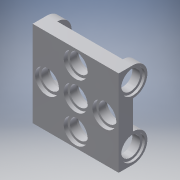
# Autodesk Inventor part: OlloHubToBase
Saved by Autodesk Inventor 2017 (Build 210142000, 142)
## iProperties
Created: 2016-06-20
Part Number: OlloHubToBase
Material: Generic
Document SubType Name: Modeling
Designer: Labtech
Density: 1 g/cm^3
Appearance: White
Author: Labtech
Autodesk Inventor part; units mm, degrees
note: some values were not read from the file. Chosen so that the rebuilt part matches the saved one: second side of "Extrusion7".
ref_plane "YZ Plane" through (0, 0, 0) normal (1, 0, 0) x (0, 1, 0)
sketch "Sketch1" plane through (0, 0, 0) normal (0, 1, 0) x (-1, 0, 0)
  line L0 (-9, 9) -> (9, 9)
  line L1 (9, 9) -> (9, -9)
  line L2 (9, -9) -> (-9, -9)
  line L3 (-9, -9) -> (-9, 9)
  line L4 (-9, 9) -> (9, -9) construction
  line L5 (9, 9) -> (-9, -9) construction
  circle A0 centre (0, 0) radius 2
  line L6 (0, 0) -> (0, -6) construction
  circle A1 centre (0, -6) radius 2
  circle A2 centre (6, 0) radius 2
  circle A3 centre (0, 6) radius 2
  circle A4 centre (-6, 0) radius 2
  dimension "d0" = 18
  dimension "d1" = 18
  dimension "d2" = 4
  dimension "d3" = 6
  dimension "d8" = 4
  dimension "d11" = 360
  constraints: 14 end point, 5 centre point, 2 coincident, 2 midpoint, 2 parallel, 1 horizontal, 1 perpendicular, 1 vertical, 9 other
  measures "d0" distance of L1.end L2.end
  measures "d1" distance of L0.end L1.end
  measures "d2" diameter of A0
  measures "d3" distance of L6.start L6.end
  measures "d8" diameter of A1
extrude "Extrusion1" add sketch "Sketch1" along normal blind 3
sketch "Sketch2" plane through (0, 3, 0) normal (0, 1, 0) x (1, 0, 0)
  circle A0 centre (0, 6) radius 2 projected
  circle A1 centre (0, 0) radius 2.5
  circle A2 centre (0, 6) radius 2.5
  circle A3 centre (-6, 0) radius 2.5
  circle A4 centre (0, -6) radius 2.5
  circle A5 centre (6, 0) radius 2.5
  dimension "d15" = 5
  dimension "d16" = 5
  dimension "d19" = 360
  constraints: 5 centre point, 2 coincident, 9 other
  measures "d15" diameter of A1
  measures "d16" diameter of A2
extrude "Extrusion2" cut sketch "Sketch2" against normal blind 0.8
sketch "Sketch3" plane through (0, 0, 0) normal (0, -1, 0) x (1, 0, 0)
  circle A0 centre (0, 0) radius 2.5
  circle A1 centre (0, -6) radius 2.5 projected
  circle A2 centre (0, -6) radius 2.5
  circle A3 centre (6, 0) radius 2.5
  circle A4 centre (0, 6) radius 2.5
  circle A5 centre (-6, 0) radius 2.5
  dimension "d25" = 360
  constraints: 5 centre point, 2 coincident, 1 concentric, 9 other
extrude "Extrusion3" cut sketch "Sketch3" against normal blind 0.8
sketch "Sketch4" plane through (9, 0, 9) normal (1, 0, 0) x (0, 0, -1)
  line L0 (0, 3) -> (3, 3) construction
  line L1 (0, 3) -> (18, 3) projected
  circle A0 centre (3, 3) radius 3
  point P0 (9, 0)
  dimension "d29" = 3
  constraints: 2 end point, 1 coincident, 1 horizontal alignment, 1 point on line, 2 other
  measures "d29" distance of L0.start L0.end
extrude "Extrusion4" add sketch "Sketch4" against normal blind 2.15
sketch "Sketch5" plane through (9, 0, 9) normal (1, 0, 0) x (0, 0, -1)
  line L0 (0, 3) -> (6, 3) projected
  arc A0 (6, 3) -> (0, 3) centre (3, 3) ccw projected
  circle A1 centre (3, 3) radius 2
  point P0 (9, 0)
  dimension "d32" = 4
  constraints: 1 centre point, 1 coincident
  measures "d32" diameter of A1
extrude "Extrusion5" cut sketch "Sketch5" against normal blind 3 contours A1 L0 | L0 A1
sketch "Sketch6" plane through (9, 0, 9) normal (1, 0, 0) x (0, 0, -1)
  circle A0 centre (3, 3) radius 2 projected
  circle A1 centre (3, 3) radius 2.5
  point P0 (9, 0)
  dimension "d35" = 5
  constraints: 1 centre point, 1 coincident
  measures "d35" diameter of A1
extrude "Extrusion6" cut sketch "Sketch6" against normal blind 0.5
sketch "Sketch7" plane through (6.85, 0, 9) normal (-1, 0, 0) x (0, 0, 1)
  arc A0 (-1, 3) -> (-5, 3) centre (-3, 3) ccw projected
  circle A1 centre (-3, 3) radius 2.5
  point P0 (-9, 0)
  dimension "d38" = 5
  constraints: 1 centre point, 1 coincident
  measures "d38" diameter of A1
extrude "Extrusion7" cut sketch "Sketch7" along normal blind 1
ref_plane "Work Plane1" through (-9, 0, 0) normal (0, 0, 1) x (1, 0, 0)
ref_plane "Work Plane2" through (0, 0, -9) normal (-1, 0, 0) x (0, 0, 1)
mirror "Mirror1" about plane through (-9, 0, 0) normal (0, 0, 1) of "Extrusion4", "Extrusion5", "Extrusion6", "Extrusion7"
mirror "Mirror2" about plane through (0, 0, -9) normal (-1, 0, 0) of "Extrusion4", "Extrusion5", "Extrusion6", "Extrusion7", "Mirror1"
body "Solid1"
